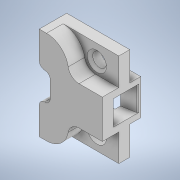
# Autodesk Inventor part: Soporte Hot End Sensor
Saved by Autodesk Inventor 2021 (Build 250183000, 183)
## iProperties
Created: 2021-08-25
Part Number: Soporte Hot End Sensor
Material: Genérico
Document SubType Name: Modeling
Designer: Diego.labarca
Density: 1 g/cm^3
Appearance: Valor por defecto
Author: Diego.labarca
Autodesk Inventor part; units mm, degrees
ref_plane "YZ Plane" through (0, 0, 0) normal (1, 0, 0) x (0, 1, 0)
ref_plane "XZ Plane" through (0, 0, 0) normal (0, 1, 0) x (-1, 0, 0)
ref_plane "XY Plane" through (0, 0, 0) normal (0, 0, 1) x (1, 0, 0)
sketch "Boceto1" plane through (0, 0, 0) normal (0, 0, 1) x (1, 0, 0)
  line L0 (-4, 8.5) -> (4, 8.5)
  line L1 (4, 8.5) -> (4, -8.5)
  line L2 (4, -8.5) -> (-4, -8.5)
  line L3 (-4, -8.5) -> (-4, 8.5)
  line L4 (0, -11.9) -> (0, 11.9) projected
  line L5 (-5.6, 0) -> (5.6, 0) projected
  point P0 (0, 0)
  dimension "d0" = 8
  dimension "d1" = 17
  constraints: 8 end point, 2 parallel, 1 horizontal, 1 perpendicular, 2 other
  measures "d0" distance of L1.end L2.end
  measures "d1" distance of L0.end L1.end
extrude "Extrusión1" add sketch "Boceto1" along normal blind 2
sketch "Boceto2" plane through (0, 0, 2) normal (0, 0, 1) x (1, 0, 0)
  circle A0 centre (0, 5.657) radius 1.25
  circle A1 centre (0, -5.657) radius 1.25
  line L0 (4, 8.5) -> (-4, 8.5) projected
  line L1 (-4, -8.5) -> (4, -8.5) projected
  point P0 (0, 0)
  dimension "d4" = 2.5
  dimension "d7" = 2.5
  dimension "d18" = 0
  dimension "d19" = 0
  dimension "d37" = 5.657
  dimension "d38" = 5.657
  constraints: 2 centre point
  measures "d4" diameter of A1
  measures "d7" diameter of A0
  measures "d18" horizontal distance of point (0, 0) A1.centre
  measures "d19" horizontal distance of A0.centre point (0, 0)
  measures "d37" distance of A0.centre point (0, 0)
  measures "d38" distance of point (0, 0) A1.centre
extrude "Extrusión2" cut sketch "Boceto2" against normal up to surface (2 mm away)
chamfer "Chaflán1" distance 0.5 angle 45 2 edges at (-1.25, 5.657, 2) (-1.25, -5.657, 2)
sketch "Boceto6" plane through (0, 0, 2) normal (0, 0, 1) x (1, 0, 0)
  line L0 (4, 8.5) -> (-4, 8.5) projected
  line L1 (-4, -8.5) -> (4, -8.5) projected
  line L2 (-4, 8.5) -> (-2.25, 8.5)
  line L3 (-2.25, 8.5) -> (-2.25, -8.5)
  line L4 (-2.25, -8.5) -> (-4, -8.5)
  line L5 (-4, -8.5) -> (-4, 8.5)
  point P0 (0, 0)
  point P1 (-0.284, 8)
  dimension "d33" = 1.75
  constraints: 8 end point, 2 parallel, 1 horizontal, 1 perpendicular, 1 point on line, 1 other
  measures "d33" distance between parallel lines of L5 L3
extrude "Extrusión6" add sketch "Boceto6" along normal blind 2
sketch "Boceto7" plane through (0, 0, 4) normal (0, 0, 1) x (1, 0, 0)
  line L0 (-4, 8.5) -> (-4, -8.5) projected
  line L1 (-4, 8.5) -> (-7.5, 8.5)
  line L2 (-7.5, 8.5) -> (-7.5, -8.5)
  line L3 (-7.5, -8.5) -> (-4, -8.5)
  line L4 (-4, -8.5) -> (-4, 8.5)
  line L5 (-9.2, 0) -> (6.2, 0) projected
  line L6 (-2.25, -8.5) -> (4, -8.5) projected
  point P0 (0, 0)
  dimension "d39" = 3.5
  constraints: 8 end point, 2 parallel, 1 collinear, 1 horizontal, 1 perpendicular, 1 point on line, 1 other
  measures "d39" distance of L3.end L2.end
extrude "Extrusión7" add sketch "Boceto7" against normal up to surface (4 mm away)
sketch "Boceto8" plane through (0, 0, 4) normal (0, 0, 1) x (1, 0, 0)
  line L0 (4, -8.5) -> (4, 8.5) projected
  line L1 (4, 3) -> (-3, 3)
  line L2 (-3, 3) -> (-3, -3)
  line L3 (-3, -3) -> (4, -3)
  line L4 (4, -3) -> (4, 3)
  line L5 (-9.8, 0) -> (6.3, 0) projected
  point P0 (0, 0)
  dimension "d43" = 7
  dimension "d44" = 6
  constraints: 8 end point, 2 parallel, 1 horizontal, 1 perpendicular, 1 point on line, 1 other
  measures "d43" distance of L3.end L2.end
  measures "d44" distance of L1.end L2.end
extrude "Extrusión8" cut sketch "Boceto8" against normal up to surface (4 mm away)
sketch "Boceto10" plane through (0, 0, 4) normal (0, 0, 1) x (1, 0, 0)
  line L0 (4, 3) -> (-3, 3) projected
  line L1 (-3, 3) -> (-4.1, 3)
  line L2 (-4.1, 3) -> (-4.1, -3)
  line L3 (-4.1, -3) -> (-3, -3)
  line L4 (-3, -3) -> (-3, 3)
  line L5 (-2.25, -3) -> (-3, -3) projected
  point P0 (0, 0)
  dimension "d51" = 1.1
  constraints: 8 end point, 2 parallel, 1 collinear, 1 horizontal, 1 perpendicular
  measures "d51" distance of L3.end L2.end
extrude "Extrusión10" cut sketch "Boceto10" against normal up to surface (4 mm away)
sketch "Boceto11" plane through (0, 0, 2) normal (0, 0, 1) x (1, 0, 0)
  line L0 (4, 3) -> (4, 8.5) projected
  line L1 (4, 3) -> (1, 3)
  line L2 (1, 3) -> (1, 2.25)
  line L3 (1, 2.25) -> (4, 2.25)
  line L4 (4, 2.25) -> (4, 3)
  point P0 (0, 0)
  dimension "d54" = 3
  dimension "d55" = 0.75
  constraints: 8 end point, 2 parallel, 1 horizontal, 1 perpendicular
  measures "d54" distance of L3.end L2.end
  measures "d55" distance of L2.end L1.end
extrude "Extrusión11" add sketch "Boceto11" against normal up to surface (2 mm away)
mirror "Simetría2" about plane through (0, 0, 0) normal (0, 1, 0) of "Extrusión11"
sketch "Boceto14" plane through (1, 2.25, 2) normal (0, -1, 0) x (1, 0, 0)
  line L0 (3, -2) -> (3, 0) projected
  line L1 (3, 0) -> (3, 1.0239)
  line L2 (3, -2) -> (-8.5, -2) projected
  line L3 (3, -2) -> (3, -3.9761)
  line L4 (0.3, -3.5) -> (0.3, 1.5)
  line L5 (3, -3.9761) -> (0.3, -3.5)
  line L6 (3, 1.0239) -> (0.3, 1.5)
  line L7 (3, -3.9761) -> (3, -3.4761)
  line L8 (3, -3.4761) -> (0.3, -3)
  line L9 (3, 1.0239) -> (3, 1.5239)
  line L10 (0.3, 1.5) -> (0.3, 2)
  line L11 (0.3, 2) -> (3, 1.5239)
  line L12 (-8.5, 2) -> (-3.25, 2) projected
  line L13 (3, 1.5239) -> (3, 2)
  line L14 (3, 2) -> (0.3, 2)
  line L15 (0.3, -3.5) -> (0.3, -4)
  line L16 (0.3, -3.5) -> (0.8, -3.5) construction
  line L17 (0.3, -4) -> (3, -4)
  line L18 (3, -4) -> (3, -3.9761)
  point P0 (-1, -2)
  point P1 (2.8356, -4)
  point P2 (0.3, -2)
  point P3 (-5, -2)
  dimension "d82" = 80
  dimension "d83" = 0.5
  dimension "d84" = 100
  dimension "d85" = 4.5
  dimension "d86" = 0.5
  dimension "d87" = 0.5
  dimension "d93" = 0
  dimension "d94" = 90
  dimension "d95" = 6
  dimension "d96" = 2.7
  constraints: 32 end point, 5 vertical, 3 perpendicular, 3 point on line, 2 horizontal, 1 parallel
  measures "d82" angle of L5 L3
  measures "d83" distance of L3.end L7.end
  measures "d84" angle of L8 L7
  measures "d85" distance of L1.end L7.end
  measures "d86" distance of L1.end L9.end
  measures "d87" distance of L4.end L10.end
  measures "d93" distance from line of L12 L10.end
  measures "d94" angle of L15 L16
  measures "d95" distance of L15.end L10.end
  measures "d96" distance between parallel lines of L4 L1
extrude "Extrusión13" add sketch "Boceto14" along normal up to surface (4.5 mm away) contours L3 L5 L4 L8 | L6 L10 L11 L9 | L18 L17 L15 L5 | L11 L14 L13
sketch "Boceto16" plane through (1.3, -2.25, 4) normal (0, -1, 0) x (1, 0, 0)
  line L0 (0, -0.5) -> (2.7, -0.9761) projected
  line L1 (2.7, -0.9761) -> (2.7, 0) projected
  line L2 (2.7, 0) -> (0, 0) projected
  line L3 (0, 0) -> (0, -0.5) projected
  line L4 (0, -6) -> (2.7, -6) projected
  line L5 (2.7, -0.9761) -> (2.7, 0) projected
  line L6 (0, -6) -> (2.7, -6)
  line L7 (2.7, -6) -> (2.7, 0)
  line L8 (2.7, 0) -> (0, 0)
  line L9 (0, 0) -> (0, -6)
  line L10 (2.7, -6) -> (2.7, -5.4761) projected
  line L11 (0, -5) -> (0, -6) projected
  line L12 (2.7, -5.4761) -> (0, -5) projected
  line L13 (0, 0) -> (0, -0.5) projected
  point P0 (-1.3, -4)
  point P1 (2.7, -0.9761)
  point P2 (2.7, -6)
  point P3 (2.7, -6)
  point P4 (2.7, -5.4761)
  point P5 (3, -5.529)
  constraints: 8 end point, 2 parallel, 1 collinear, 1 horizontal, 1 perpendicular
extrude "Extrusión15" add sketch "Boceto16" along normal blind 1
mirror "Simetría4" about plane through (0, 0, 0) normal (0, 1, 0) of "Extrusión15"
fillet "Empalme6" radius 0.2 1 edges at (4, 0, -1.4761)
sketch "Boceto18" plane through (0, 0, 4) normal (0, 0, 1) x (1, 0, 0)
  line L0 (-2.25, -8.5) -> (-2.25, -3) projected
  line L1 (4, 2.25) -> (4, -8.5) projected
  line L2 (-2.25, -3) -> (4, -3)
  line L3 (4, -3) -> (4, -3.5)
  line L4 (4, -3.5) -> (-2.25, -3.5)
  line L5 (-2.25, -3.5) -> (-2.25, -3)
  line L6 (-2.25, 3) -> (1, 3) projected
  line L7 (4, 2.25) -> (4, 8.5) projected
  line L8 (-2.25, 3) -> (4, 3)
  line L9 (4, 3) -> (4, 3.5)
  line L10 (4, 3.5) -> (-2.25, 3.5)
  line L11 (-2.25, 3.5) -> (-2.25, 3)
  point P0 (0, 0)
  point P1 (4, -3.25)
  point P2 (4, 3.25)
  point P3 (-2.25, -3.5)
  point P4 (4, -3)
  point P5 (1, 3)
  point P6 (4, 3)
  point P7 (4, -3)
  dimension "d102" = 0.5
  dimension "d103" = 0.5
  constraints: 16 end point, 4 parallel, 2 horizontal, 2 perpendicular, 2 point on line
  measures "d102" distance of L2.end L3.end
  measures "d103" distance of L9.end L8.end
extrude "Extrusión16" add sketch "Boceto18" against normal up to surface (2 mm away)
fillet "Empalme7" radius 2 2 edges at (-2.25, -3.5, 3) (-2.25, 3.5, 3)
fillet "Empalme8" radius 1 2 edges at (1, 3, 1) (1, -3, 1)
fillet "Empalme9" radius 4 2 edges at (-2.25, 8.5, 3) (-2.25, -8.5, 3)
sketch "Boceto19" plane through (0, 0, 4) normal (0, 0, 1) x (1, 0, 0)
  line L0 (-4.1, -3) -> (1.3, -3) projected
  line L1 (-4.1, -3) -> (-4.1, 3) projected
  line L2 (-4.1, 3) -> (1.3, 3) projected
  line L3 (1.3, 3) -> (1.3, -3) projected
  arc A0 (-6.1661, -8.5) -> (-2.222, -5.1667) centre (-6.1661, -4.5) ccw projected
  arc A1 (-0.25, -3.5) -> (-2.222, -5.1667) centre (-0.25, -5.5) ccw projected
  line L4 (4, -3.5) -> (-0.25, -3.5) projected
  line L5 (4, 3.5) -> (4, -3.5) projected
  line L6 (4, 3.5) -> (-0.25, 3.5) projected
  arc A2 (-2.222, 5.1667) -> (-0.25, 3.5) centre (-0.25, 5.5) ccw projected
  arc A3 (-2.222, 5.1667) -> (-6.1661, 8.5) centre (-6.1661, 4.5) ccw projected
  line L7 (-7.5, 8.5) -> (-7.5, -8.5) projected
  line L8 (-6.1661, 8.5) -> (-7.5, 8.5) projected
  line L9 (-7.5, -8.5) -> (-6.1661, -8.5) projected
  point P0 (0, 0)
extrude "Extrusión17" add sketch "Boceto19" along normal blind 1 contours L1 L2 L3 L0 | L9 L7 L8 A3 A2 L6 L5 L4 A1 A0
sketch "Boceto20" plane through (0, 0, 5) normal (0, 0, 1) x (1, 0, 0)
  line L0 (-7.5, -8.5) -> (-7.5, 8.5) projected
  line L1 (-7.5, 2.5) -> (-5.5, 2.5)
  line L2 (-5.5, 2.5) -> (-5.5, -2.5)
  line L3 (-5.5, -2.5) -> (-7.5, -2.5)
  line L4 (-7.5, -2.5) -> (-7.5, 2.5)
  line L5 (-9.8, 0) -> (6.3, 0) projected
  point P0 (0, 0)
  dimension "d111" = 2
  dimension "d112" = 5
  constraints: 8 end point, 2 parallel, 1 horizontal, 1 perpendicular, 1 point on line, 1 other
  measures "d111" distance of L2.end L3.end
  measures "d112" distance of L1.end L2.end
extrude "Extrusión18" cut sketch "Boceto20" against normal up to surface (5 mm away)
fillet "Empalme10" radius 1 4 edges at (-7.5, 2.5, 2.5) (-7.5, -2.5, 2.5) (-5.5, 2.5, 2.5) (-5.5, -2.5, 2.5)
equation "\"d4\" = d7"
equation "\"d38\" = d37"
equation "\"d86\" = d83"
equation "\"d87\" = d86"
